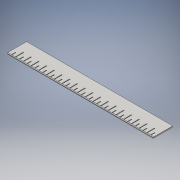
# Autodesk Inventor part: ruler
Saved by Autodesk Inventor 2016 (Build 200138000, 138)
## iProperties
Created: 2016-08-27
Part Number: ruler
Material: Generic
Document SubType Name: Modeling
Designer: Administrator
Density: 1 g/cm^3
Appearance: Default
Author: Administrator
Autodesk Inventor part; units mm, degrees
ref_plane "YZ Plane" through (0, 0, 0) normal (1, 0, 0) x (0, 1, 0)
ref_plane "XZ Plane" through (0, 0, 0) normal (0, 1, 0) x (-1, 0, 0)
ref_plane "XY Plane" through (0, 0, 0) normal (0, 0, 1) x (1, 0, 0)
sketch "Sketch1" plane through (0, 0, 0) normal (0, 0, 1) x (1, 0, 0)
  line L0 (-37.8, 0) -> (226.8, 0) projected
  line L1 (0, -5) -> (0, 30) projected
  line L2 (0, 0) -> (189, 0)
  line L3 (189, 0) -> (189, 25)
  line L4 (189, 25) -> (0, 25)
  line L5 (0, 25) -> (0, 0)
  dimension "d0" = 189
  dimension "d1" = 25
  constraints: 8 end point, 2 parallel, 1 horizontal, 1 perpendicular
  measures "d0" distance of L4.end L3.end
  measures "d1" distance of L3.end L2.end
extrude "Extrusion1" add sketch "Sketch1" along normal blind 1.5
sketch "Sketch6" plane through (0, 0, 0) normal (-1, 0, 0) x (0, 0, 1)
  line L0 (0, 25) -> (0, 0) projected
  line L1 (0, 0) -> (1.5, 0) projected
  line L2 (1.5, 25) -> (1.5, 0) projected
  line L3 (0, 25) -> (1.5, 25) projected
  line L4 (0, 0) -> (1.5, 0) projected
  line L5 (1.5, 0) -> (0.75, 0)
  line L6 (0.75, 0) -> (1.5, 0.75)
  line L7 (0.75, 0) -> (1.2803, 0) construction
  line L8 (1.5, 0.75) -> (1.5, 0)
  line L9 (0, 0) -> (1.5, 0) projected
  point P0 (0.75, 0)
  dimension "d42" = 45
  constraints: 8 end point, 3 midpoint, 1 horizontal, 1 point on line, 1 vertical
  measures "d42" angle of L7 L6
extrude "Extrusion6" cut sketch "Sketch6" against normal through all contours L6 L2 L1
sketch "Sketch7" plane through (0, 0, 1.5) normal (0, 0, 1) x (1, 0, 0)
  line L0 (0, 0.75) -> (189, 0.75) projected
  line L1 (189, 0.75) -> (189, 25) projected
  line L2 (189, 25) -> (0, 25) projected
  line L3 (0, 25) -> (0, 0.75) projected
  line L4 (0, 0.75) -> (189, 0.75) projected
  line L5 (4.6, 0.75) -> (5.4, 0.75)
  line L6 (5.4, 0.75) -> (5.4, 5.75)
  line L7 (5.4, 5.75) -> (4.6, 5.75)
  line L8 (4.6, 5.75) -> (4.6, 0.75)
  line L9 (5, 5.75) -> (5, 6.75) construction
  line L10 (9.6, 0.75) -> (10.4, 0.75)
  line L11 (10.4, 0.75) -> (10.4, 10.75)
  line L12 (10.4, 10.75) -> (9.6, 10.75)
  line L13 (9.6, 10.75) -> (9.6, 0.75)
  line L14 (10, 10.75) -> (10, 11.75) construction
  point P0 (0, 0)
  dimension "d45" = 0.8
  dimension "d46" = 5
  dimension "d47" = 1
  dimension "d48" = 5
  dimension "d49" = 0.8
  dimension "d50" = 10
  dimension "d51" = 1
  dimension "d52" = 5
  constraints: 20 end point, 4 parallel, 2 horizontal, 2 midpoint, 2 perpendicular, 2 point on line, 2 vertical
  measures "d45" distance of L7.end L6.end
  measures "d46" distance of L6.end L5.end
  measures "d47" distance of L9.start L9.end
  measures "d48" distance from line of L3 L9.start
  measures "d49" distance of L12.end L11.end
  measures "d50" distance of L11.end L10.end
  measures "d51" distance of L14.start L14.end
  measures "d52" horizontal distance of L14.start L9.start
extrude "Extrusion7" cut sketch "Sketch7" against normal blind 0.6 contours L8 L7 L6 L0 | L13 L12 L11 L0
pattern_linear "Rectangular Pattern3" count 19 spacing 10 along (1, 0, 0) of "Extrusion7"
body "Solid1"
